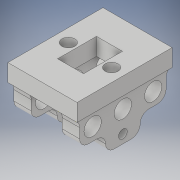
# Autodesk Inventor part: Y_Slider_Part
Saved by Autodesk Inventor 2019 (Build 230136000, 136)
## iProperties
Created: 2018-08-19
Part Number: Y_Slider_Part
Material: Generic
Document SubType Name: Modeling
Designer: Julia
Density: 1 g/cm^3
Appearance: Default
Author: Julia
Autodesk Inventor part; units mm, degrees
ref_plane "YZ Plane" through (0, 0, 0) normal (1, 0, 0) x (0, 1, 0)
ref_plane "XZ Plane" through (0, 0, 0) normal (0, 1, 0) x (-1, 0, 0)
ref_plane "XY Plane" through (0, 0, 0) normal (0, 0, 1) x (1, 0, 0)
sketch "Sketch1" plane through (0, 0, 0) normal (0, 1, 0) x (-1, 0, 0)
  line L0 (40, 55) -> (-40, 55)
  line L1 (-40, 55) -> (-40, -55)
  line L2 (-40, -55) -> (40, -55)
  line L3 (40, -55) -> (40, 55)
  point P0 (0, 0)
  point P1 (40, 0)
  point P2 (0, 55)
  dimension "d0" = 110
  dimension "d1" = 80
  constraints: 8 end point, 2 midpoint, 2 parallel, 1 horizontal, 1 horizontal alignment, 1 perpendicular, 1 vertical alignment
  measures "d0" distance of L2.end L0.start
  measures "d1" distance of L1.end L2.end
extrude "Extrusion1" add sketch "Sketch1" along normal blind 20
sketch "Sketch2" plane through (0, 0, 0) normal (0, -1, 0) x (1, 0, 0)
  line L0 (38, 50) -> (18, 50)
  line L1 (18, 50) -> (18, 20)
  line L2 (18, 20) -> (38, 20)
  line L3 (38, 20) -> (38, 50)
  line L4 (40, 55) -> (40, -55) projected
  line L5 (-18, 50) -> (-38, 50)
  line L6 (-38, 50) -> (-38, 20)
  line L7 (-38, 20) -> (-18, 20)
  line L8 (-18, 20) -> (-18, 50)
  line L9 (-40, -55) -> (-40, 55) projected
  line L10 (47.026, 0) -> (-61.5148, 0) construction
  line L11 (38, -50) -> (18, -50)
  line L12 (18, -50) -> (18, -20)
  line L13 (18, -20) -> (38, -20)
  line L14 (38, -20) -> (38, -50)
  line L15 (-18, -50) -> (-38, -50)
  line L16 (-38, -50) -> (-38, -20)
  line L17 (-38, -20) -> (-18, -20)
  line L18 (-18, -20) -> (-18, -50)
  point P0 (0, 0)
  dimension "d4" = 30
  dimension "d5" = 20
  dimension "d6" = 20
  dimension "d7" = 2
  dimension "d8" = 20
  dimension "d9" = 2
  constraints: 34 end point, 8 symmetric about line, 4 horizontal, 4 parallel, 2 collinear, 2 perpendicular
  measures "d4" distance of L2.end L0.start
  measures "d5" distance of L0.start L0.end
  measures "d6" vertical distance of L1.end point (0, 0)
  measures "d7" distance between parallel lines of L4 L3
  measures "d8" distance of L5.start L5.end
  measures "d9" distance between parallel lines of L9 L6
extrude "Extrusion2" add sketch "Sketch2" along normal blind 30
sketch "Sketch3" plane through (38, 0, 50) normal (1, 0, 0) x (0, 0, -1)
  line L0 (30, -30) -> (0, -30) projected
  line L1 (30, 0) -> (30, -30) projected
  line L2 (100, 0) -> (100, -30) projected
  line L3 (100, -30) -> (70, -30) projected
  point P0 (50, 0)
  point P1 (15, -15)
  point P2 (15, -30)
  point P3 (30, -15)
  point P4 (85, -15)
  point P5 (100, -15)
  point P6 (85, -30)
  constraints: 4 midpoint, 2 horizontal alignment, 2 vertical alignment
hole "Hole1" at (38, -15, 35) at (38, -15, -35) direction (-1, 0, 0) diameter 20 end through all
sketch "Sketch4" plane through (0, 20, 0) normal (0, 1, 0) x (1, 0, 0)
  circle A0 centre (25, 0) radius 7.5
  circle A1 centre (-25, 0) radius 7.5
  point P0 (0, 0)
  dimension "d19" = 15
  dimension "d20" = 15
  dimension "d21" = 25
  dimension "d23" = 25
  constraints: 2 centre point, 2 horizontal alignment
  measures "d19" diameter of A0
  measures "d20" diameter of A1
  measures "d21" distance of point (0, 0) A0.centre
  measures "d23" distance of point (0, 0) A1.centre
extrude "Extrusion3" cut sketch "Sketch4" against normal blind 15
fillet "Fillet1" radius 10 4 edges at (28, 0, 50) (-28, 0, 50) (-28, 0, -50) (28, 0, -50)
fillet "Fillet3" radius 10 4 edges at (28, -30, 50) (-28, -30, 50) (-28, -30, -50) (28, -30, -50)
sketch "Sketch5" plane through (0, 20, 0) normal (0, 1, 0) x (1, 0, 0)
  line L0 (15, 22.5) -> (-15, 22.5)
  line L1 (-15, 22.5) -> (-15, -22.5)
  line L2 (-15, -22.5) -> (15, -22.5)
  line L3 (15, -22.5) -> (15, 22.5)
  point P0 (0, 0)
  point P1 (15, 0)
  point P2 (0, 22.5)
  dimension "d30" = 45
  dimension "d31" = 30
  constraints: 8 end point, 2 midpoint, 2 parallel, 1 horizontal, 1 horizontal alignment, 1 perpendicular, 1 vertical alignment
  measures "d30" distance of L2.end L0.start
  measures "d31" distance of L1.end L2.end
extrude "Extrusion4" cut sketch "Sketch5" against normal blind 20
sketch "Sketch6" plane through (0, 0, 0) normal (0, -1, 0) x (1, 0, 0)
  line L0 (38, 20) -> (18, 20)
  line L1 (18, 20) -> (18, -20)
  line L2 (18, -20) -> (38, -20)
  line L3 (38, -20) -> (38, 20)
  line L4 (38, 55) -> (38, 20) projected
  line L5 (18, 20) -> (18, 55) projected
  line L6 (38, 20) -> (18, 20) projected
  line L7 (18, -20) -> (38, -20) projected
  line L8 (-18, 20) -> (-38, 20)
  line L9 (-38, 20) -> (-38, -20)
  line L10 (-38, -20) -> (-18, -20)
  line L11 (-18, -20) -> (-18, 20)
  line L12 (-38, -55) -> (-38, -20) projected
  line L13 (-38, -20) -> (-18, -20) projected
  line L14 (-18, -20) -> (-18, -55) projected
  line L15 (-18, 20) -> (-38, 20) projected
  point P0 (0, 0)
  constraints: 16 end point, 8 collinear, 4 parallel, 2 horizontal, 2 perpendicular
extrude "Extrusion6" add sketch "Sketch6" along normal blind 50 contours L11 L10 L9 L8
extrude "Extrusion7" add sketch "Sketch6" along normal blind 50 contours L3 L2 L1 L0
sketch "Sketch7" plane through (38, 0, 55) normal (1, 0, 0) x (0, 0, -1)
  circle A0 centre (55, -15) radius 10
  line L0 (0, 0) -> (110, 0) projected
  line L1 (0, 0) -> (110, 0) projected
  point P0 (55, 0)
  point P1 (55, 0)
  dimension "d42" = 20
  dimension "d43" = 15
  constraints: 1 centre point, 1 midpoint, 1 vertical alignment
  measures "d42" diameter of A0
  measures "d43" distance from line of A0.centre L0
extrude "Extrusion8" cut sketch "Sketch7" against normal blind 100
sketch "Sketch9" plane through (38, 0, 55) normal (1, 0, 0) x (0, 0, -1)
  circle A0 centre (55, -40) radius 5
  line L0 (75, -50) -> (35, -50) projected
  line L1 (95, -30) -> (75, -30) projected
  point P0 (55, 0)
  point P1 (55, -50)
  dimension "d46" = 10
  dimension "d47" = 10
  constraints: 1 centre point, 1 midpoint, 1 vertical alignment
  measures "d46" diameter of A0
  measures "d47" distance from line of L1 A0.centre
extrude "Extrusion9" cut sketch "Sketch9" against normal blind 100
fillet "Fillet7" radius 10 4 edges at (-28, -50, 20) (28, -50, 20) (28, -50, -20) (-28, -50, -20)
fillet "Fillet8" radius 10 4 edges at (28, -30, -20) (-28, -30, -20) (28, -30, 20) (-28, -30, 20)
body "Solid1"
